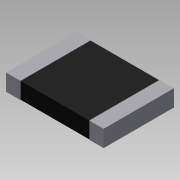
# Autodesk Inventor part: GP-WSM010
Saved by Autodesk Inventor 2011 (Build 150239000, 239)
## iProperties
Created: 2010-11-25
Part Number: GP-WSM010
Document SubType Name: Modeling
Designer: abbath
Density: 1 g/cm^3
Mass: 0.012785 g
Surface Area: 0.45347 cm^2
Volume: 0.012785 cm^3
Author: abbath
Autodesk Inventor part; units mm, degrees
ref_plane "YZ Plane" through (0, 0, 0) normal (1, 0, 0) x (0, 1, 0)
ref_plane "XZ Plane" through (0, 0, 0) normal (0, 1, 0) x (-1, 0, 0)
ref_plane "XY Plane" through (0, 0, 0) normal (0, 0, 1) x (1, 0, 0)
sketch "Эскиз1" plane through (0, 0, 0) normal (0, 0, 1) x (1, 0, 0)
  line L0 (-2.365, 1.705) -> (2.365, 1.705)
  line L1 (2.365, 1.705) -> (2.365, -1.705)
  line L2 (2.365, -1.705) -> (-2.365, -1.705)
  line L3 (-2.365, -1.705) -> (-2.365, 1.705)
  point P0 (0, 0)
  dimension "d0" = 3.41
  dimension "d1" = 4.73
  dimension "d2" = 2.365
  dimension "d3" = 1.705
  constraints: 8 end point, 2 parallel, 1 horizontal, 1 perpendicular
  measures "d0" distance between parallel lines of L2 L0
  measures "d1" distance between parallel lines of L1 L3
  measures "d2" distance from line of L3 point (0, 0)
  measures "d3" distance from line of L0 point (0, 0)
extrude "Выдавливание1" add sketch "Эскиз1" along normal blind 0.81
sketch "Эскиз2" plane through (0, 0, 0.81) normal (0, 0, 1) x (1, 0, 0)
  line L0 (2.365, 1.705) -> (2.365, -1.705) projected
  line L1 (-2.365, 1.705) -> (2.365, 1.705) projected
  line L2 (-2.365, -1.705) -> (-2.365, 1.705) projected
  line L3 (2.365, -1.705) -> (-2.365, -1.705) projected
  line L4 (-1.665, 1.705) -> (1.665, 1.705)
  line L5 (1.665, 1.705) -> (1.665, -1.705)
  line L6 (1.665, -1.705) -> (-1.665, -1.705)
  line L7 (-1.665, -1.705) -> (-1.665, 1.705)
  point P0 (0, 0)
  dimension "d6" = 0.7
  dimension "d7" = 0.7
  constraints: 8 end point, 2 collinear, 2 parallel, 1 horizontal, 1 perpendicular
  measures "d6" distance between parallel lines of L2 L7
  measures "d7" distance between parallel lines of L0 L5
extrude "Выдавливание2" cut sketch "Эскиз2" against normal blind 0.01 contours L5 L3 L7 L1
sketch "Эскиз3" plane through (-2.365, -1.705, 0) normal (0, -1, 0) x (1, 0, 0)
  line L0 (4.73, 0) -> (0, 0) projected
  line L1 (4.03, 0.8) -> (0.7, 0.8) projected
  line L2 (0.7, 0.8) -> (0.7, 0)
  line L3 (4.03, 0.8) -> (4.03, 0)
  point P0 (2.365, 0)
  constraints: 4 end point, 2 perpendicular, 2 point on line
extrude "Выдавливание3" cut sketch "Эскиз3" against normal blind 0.01
sketch "Эскиз4" plane through (0, 0, 0) normal (0, 0, -1) x (-1, 0, 0)
  line L0 (-1.665, -1.695) -> (1.665, -1.695) projected
  line L1 (2.365, 1.705) -> (-2.365, 1.705) projected
  line L2 (1.665, -1.695) -> (1.665, 1.705)
  line L3 (-1.665, -1.695) -> (-1.665, 1.705)
  point P0 (0, 0)
  constraints: 4 end point, 2 perpendicular, 2 point on line
extrude "Выдавливание4" cut sketch "Эскиз4" against normal blind 0.01
sketch "Эскиз5" plane through (-2.365, 1.705, 0.81) normal (0, 1, 0) x (1, 0, 0)
  line L0 (0.7, 0.01) -> (4.03, 0.01) projected
  line L1 (4.03, 0.8) -> (0.7, 0.8) projected
  line L2 (4.03, 0.01) -> (4.03, 0.8)
  line L3 (0.7, 0.01) -> (0.7, 0.8)
  point P0 (2.365, 0.81)
  constraints: 4 end point, 2 perpendicular
extrude "Выдавливание5" cut sketch "Эскиз5" against normal blind 0.01
equation "\"d2\" = 0.5 * d1"
equation "\"d3\" = 0.5 * d0"
equation "\"d7\" = d6"
